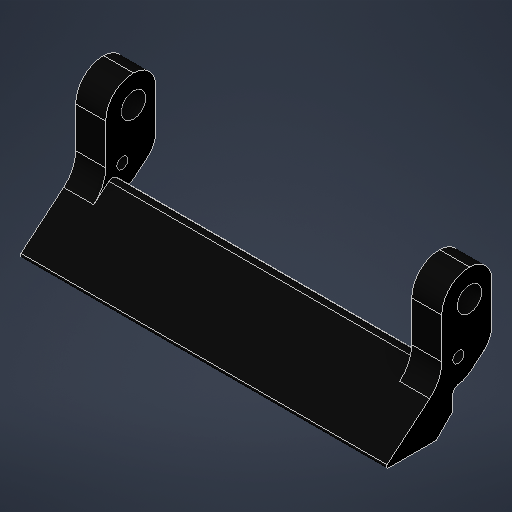
# Autodesk Inventor part: Schaufel
Saved by Autodesk Inventor 2025.2 (Build 292293000, 293)
## iProperties
Part Number: Schaufel
Material: Aluminium 6061
Document SubType Name: Modeling
Designer: rYan
Mass: 10.967 g
Surface Area: 30.2735 cm^2
Volume: 4.06184 cm^3
Density: 2.7 g/cm^3
Appearance: Vorgabe
Author: rYan
Autodesk Inventor part; units mm, degrees
ref_plane "YZ Plane" through (0, 0, 0) normal (1, 0, 0) x (0, 1, 0)
ref_plane "XZ Plane" through (0, 0, 0) normal (0, 1, 0) x (-1, 0, 0)
ref_plane "XY Plane" through (0, 0, 0) normal (0, 0, 1) x (1, 0, 0)
sketch "Skizze1" plane through (0, 0, 0) normal (1, 0, 0) x (0, 1, 0)
  line L0 (-4.1616, 7.0772) -> (-12, 0.5)
  line L1 (-12, 0) -> (-3, 0)
  line L2 (-12, 0.5) -> (-12, 0)
  line L3 (0, 5) -> (8, 11.7128)
  circle A0 centre (3, 19) radius 0.5
  line L4 (-2, 11.7128) -> (-2, 24)
  line L5 (-2, 24) -> (8, 24)
  line L6 (8, 24) -> (8, 11.7128)
  line L7 (0, 3) -> (-3, 0)
  line L8 (8, 11.7128) -> (-2, 11.7128) construction
  arc A1 (-4.1616, 7.0772) -> (-2, 11.7128) centre (-8.0514, 11.7128) ccw
  line L9 (0, 5) -> (0, 3)
  line L10 (3, 19) -> (3, 0) construction
  point P0 (0, 0)
  dimension "d40" = 0.5
  dimension "d44" = 1
  dimension "d59" = 10
  dimension "d60" = 45
  dimension "d61" = 5
  dimension "d63" = 40
  dimension "d78" = 3
  dimension "d79" = 12
  dimension "d80" = 0
  dimension "d81" = 19
  dimension "d82" = 5
  dimension "d83" = 3
  constraints: 22 end point, 5 vertical, 2 centre point, 2 horizontal, 2 point on circle, 2 tangent, 1 parallel, 1 perpendicular, 1 point on line, 1 other
  measures "d40" distance of L0.end L1.start
  measures "d44" diameter of A0
  measures "d59" distance of L4.end L5.end
  measures "d60" angle of L7 L1
  measures "d61" distance from line of L3.start L1
  measures "d63" angle of L0 L1
  measures "d78" distance of point (0, 0) L1.end
  measures "d79" distance from line of point (0, 0) L2
  measures "d80" distance from line of point (0, 0) L9
  measures "d81" vertical distance of point (0, 0) L10.start
  measures "d82" distance from line of L5 L10.start
  measures "d83" horizontal distance of point (0, 0) L10.start
extrude "Extrusion1" add sketch "Skizze1" along normal mid plane 67
sketch "Skizze6" plane through (0, 0, 0) normal (0, 1, 0) x (-1, 0, 0)
  line L0 (33.5, 0.5) -> (-33.5, 0.5) projected
  line L1 (-33.5, 7.0772) -> (-33.5, 0.5) projected
  line L2 (33.5, 0.5) -> (33.5, 7.0772) projected
  line L3 (-27.5, 6) -> (27.5, 6)
  line L4 (27.5, 6) -> (27.5, 31)
  line L5 (27.5, 31) -> (-27.5, 31)
  line L6 (-27.5, 31) -> (-27.5, 6)
  line L7 (0, -6.2) -> (0, 37.2) projected
  line L8 (33.5, 0) -> (-33.5, 0) projected
  line L9 (-33.5, 0) -> (33.5, 0) projected
  point P0 (0, 0)
  point P1 (-33, 10)
  point P2 (33, 10)
  dimension "d45" = 6
  dimension "d46" = 25
  dimension "d50" = 6
  constraints: 8 end point, 2 parallel, 1 horizontal, 1 perpendicular, 3 other
  measures "d46" distance of L3.end L4.end
  measures "d50" distance between parallel lines of L8 L3
extrude "Extrusion4" cut sketch "Skizze6" along normal mid plane 16
sketch "Skizze3" plane through (-33.5, 0, 0) normal (-1, 0, 0) x (0, 0, 1)
  line L0 (0, -3) -> (0, -12) projected
  line L1 (0.5, -12) -> (7.0772, -4.1616) projected
  line L2 (0, -12) -> (0, 0) construction
  line L3 (0, 12) -> (0, -16) projected
  line L4 (0, -12) -> (0.5, -12) projected
  line L5 (11.7128, 8) -> (5, 0) projected
  line L6 (11.7128, -2) -> (24, -2) projected
  line L7 (24, -2) -> (24, 8) projected
  line L8 (24, 8) -> (11.7128, 8) projected
  circle A0 centre (19, 3) radius 0.5 projected
  line L9 (3, 0) -> (0, -3) projected
  arc A1 (11.7128, -2) -> (7.0772, -4.1616) centre (11.7128, -8.0514) ccw projected
  line L10 (5, 0) -> (3, 0) projected
  constraints: 1 coincident
hole "Bohrung1" at (-33.5, 3, 19) direction (1, 0, 0) diameter 4.4 end through all
sketch "Skizze4" plane through (-33.5, 0, 0) normal (-1, 0, 0) x (0, 0, 1)
  line L0 (0, 12) -> (0, -16) projected
  line L1 (-5.8, 0) -> (34.8, 0) projected
  point P0 (29, 0)
  point P1 (11, 1)
  dimension "d38" = 11
  dimension "d84" = 1
  measures "d38" distance from line of point (11, 1) L0
  measures "d84" distance from line of point (11, 1) L1
hole "Bohrung2" at (-33.5, 1, 11) direction (1, 0, 0) diameter 2 end through all
fillet "Rundung2" radius 5 6 edges at (30.5, -2, 24) (30.5, 8, 24) (-30.5, 8, 24) (-30.5, -2, 24) (30.5, 8, 11.7128) (-30.5, 8, 11.7128)
fillet "Rundung8" radius 0.36 2 edges at (0, -12, 0.5) (0, -12, 0)
sketch "Skizze7" plane through (-27.5, 1.1918, 6) normal (0, 0, 1) x (1, 0, 0)
  line L0 (0, 0) -> (55, 0) projected
  line L1 (0, 0) -> (0, -6.6371) projected
  line L2 (55, -6.6371) -> (0, -6.6371) projected
  line L3 (55, -6.6371) -> (55, 0) projected
  line L4 (-19.4, -1.1918) -> (74.4, -1.1918) projected
  point P0 (27.5, -1.1918)
  point P1 (0, -1.1918)
  point P2 (55, -1.1918)
extrude "Extrusion5" cut sketch "Skizze7" against normal through all contours L0 L3 L4 L1
sketch "Skizze8" plane through (-27.5, -5.4454, 6) normal (1, 0, 0) x (0, 0, -1)
  line L0 (-8.0443, 13.4454) -> (-13, 13.4454) projected
  line L1 (-10.5222, 13.4454) -> (-10.5222, 12.4454)
  line L2 (-10.5222, 12.4454) -> (-17.4656, 12.4454)
  line L3 (-17.4656, 12.4454) -> (-4.9838, 12.4454)
  line L4 (-4.9838, 12.4454) -> (-4.9838, 14.4351)
  line L5 (-4.9838, 14.4351) -> (-17.4656, 14.4351)
  line L6 (-17.4656, 14.4351) -> (-17.4656, 12.4454)
  point P0 (6, 5.4454)
  dimension "d90" = 1
  constraints: 12 end point, 2 parallel, 2 perpendicular, 1 horizontal, 1 midpoint, 1 vertical
  measures "d90" distance of L1.start L1.end
extrude "Extrusion6" cut sketch "Skizze8" along normal mid plane 200
fillet "Rundung10" radius 4 4 edges at (30.5, 7, 11.0443) (30.5, 7, 22.0001) (-30.5, 7, 22.0001) (-30.5, 7, 11.0443)
sketch "Skizze9" plane through (-27.5, -2, 19) normal (1, 0, 0) x (0, 0, -1)
  line L0 (9.3252, 7.5712) -> (14, 2) projected
  line L1 (14, 2) -> (14, 3)
  line L2 (14, 3) -> (12.8, 3)
  line L3 (12.8, 3) -> (14, 3)
  line L4 (14, 3) -> (14, 4.2192)
  line L5 (14, 4.2192) -> (12.8, 4.2192)
  line L6 (12.8, 4.2192) -> (12.8, 3)
  line L7 (12.3, 4.7192) -> (14.5, 4.7192)
  line L8 (14.5, 4.7192) -> (14.5, 2.5)
  line L9 (14.5, 2.5) -> (12.3, 2.5)
  line L10 (12.3, 2.5) -> (12.3, 4.7192)
  line L11 (12.3, 2.5) -> (12.3, 1.2569)
  line L12 (12.3, 1.2569) -> (14.6235, 1.2569)
  line L13 (12.3, 1.2569) -> (11.55, 1.2569)
  line L14 (11.55, 1.2569) -> (11.55, 4.7192)
  line L15 (11.55, 4.7192) -> (12.3, 4.7192)
  point P0 (19, 2)
  point P1 (13.5805, 2.5)
  point P2 (12.3, 4.026)
  point P3 (11.55, 4.45)
  point P4 (13.1609, 3)
  point P5 (14, 2.5)
  dimension "d95" = 1
  dimension "d96" = 1.2
  dimension "d97" = 0.5
  dimension "d103" = 0.75
  constraints: 30 end point, 6 perpendicular, 4 parallel, 2 horizontal, 2 vertical, 1 point on line, 3 other
  measures "d95" distance of L0.end L1.end
  measures "d96" distance of L1.end L2.end
  measures "d97" distance between parallel lines of L5 L7
  measures "d103" distance of L11.end L13.end
extrude "Extrusion7" cut sketch "Skizze9" along normal mid plane 200 contours L10 L7 L8 L9 L1 L4 L5 L6 L0 | L0 L6 L2 L9 L10 | L6 L5 L4 L2 L0 | L0 L2 L6 | L2 L1 L9 L0 | L9 L1 L0
fillet "Rundung12" radius 4 2 edges at (30.5, 2.026, 6.7) (-30.5, 2.026, 6.7)
sketch "Skizze16" plane through (-27.5, 0, 6) normal (0, 0, 1) x (1, 0, 0)
  line L0 (27.5, 0) -> (27.5, -5.4454)
  line L1 (55, -5.4454) -> (0, -5.4454) projected
  line L2 (27.5, -5.4454) -> (27.5, -26.9454)
  circle A0 centre (27.5, -26.9454) radius 21.5
  circle A1 centre (27.5, -26.9454) radius 24.5
  line L3 (0, -5.4454) -> (0, 0)
  line L4 (-6, 0) -> (61, 0) projected
  line L5 (0, 0) -> (55, 0)
  line L6 (55, 0) -> (55, -5.4454)
  line L7 (55, -5.4454) -> (0, -5.4454)
  line L8 (0, -5.4454) -> (0, 0)
  point P0 (15.7527, -5.4454)
  point P1 (39.2473, -5.4454)
  point P2 (55, 0)
  dimension "d122" = 21.5
  dimension "d123" = 3
  constraints: 14 end point, 2 parallel, 2 point on line, 1 centre point, 1 coincident, 1 horizontal, 1 midpoint, 1 perpendicular, 1 vertical, 1 vertical alignment, 2 other
  measures "d122" distance of L0.end L2.end
extrude "Extrusion11" add sketch "Skizze16" along normal blind 5 contours L4 L6 L1 A1 L0 | L0 A1 L1 L3 L4 | A1 L1 L0 | L0 L1 A1
sketch "Skizze18" plane through (27.5, -5.4454, 11) normal (1, 0, 0) x (0, 0, -1)
  line L0 (10.3642, -6.3928) -> (3.9228, 1.2837) projected
  line L1 (10.3642, -6.3928) -> (0, 5.9588)
  line L2 (0, 0) -> (0, 3.4032) projected
  line L3 (0, 5.9588) -> (0, 0)
  line L4 (0, 0) -> (5, 0)
  point P0 (11, 5.4454)
  point P1 (5, 0)
  constraints: 6 end point, 2 collinear, 1 perpendicular, 1 point on line
extrude "Extrusion12" cut sketch "Skizze18" against normal up to surface (55 mm away)
sketch "Skizze19" plane through (27.5, -2, 11.7128) normal (-1, 0, 0) x (0, 0, 1)
  circle A0 centre (-0.7128, 3) radius 1 projected
  circle A1 centre (-0.7128, 3) radius 2
  point P0 (-11.7128, 2)
  dimension "d131" = 4
  constraints: 1 centre point, 1 coincident
  measures "d131" diameter of A1
extrude "Extrusion13" cut sketch "Skizze19" along normal up to surface (55 mm away) contours A0 | A1
sketch "Skizze22" plane through (33.5, 0, 0) normal (1, 0, 0) x (0, 0, -1)
  line L0 (0, -3) -> (-3, 0) projected
  line L1 (-5.4195, 0.5) -> (-6.7, 0.5) projected
  line L2 (-3, 0) -> (-6.7, 0)
  line L3 (-6.7, 0) -> (-6.7, 0.5)
  line L4 (-6.7, 0.5) -> (-3, 0.5)
  line L5 (-3, 0.5) -> (-3, 0)
  point P0 (0, 0)
  point P1 (-5.4195, 0.5)
  constraints: 8 end point, 2 parallel, 1 horizontal, 1 perpendicular
extrude "Extrusion14" cut sketch "Skizze22" against normal up to surface (67 mm away)
fillet "Rundung22" radius 1 2 edges at (30.5, 0, 6.7) (-30.5, 0, 6.7)
sketch "Skizze23" plane through (-33.5, -2, 11.7128) normal (0, -1, 0) x (1, 0, 0)
  line L0 (0, 8.2872) -> (0, 12.2872) projected
  line L1 (0, 12.2872) -> (67, 12.2872)
  line L2 (67, 12.2872) -> (67, -11.7128)
  line L3 (67, -11.7128) -> (0, -11.7128)
  line L4 (0, -11.7128) -> (0, 12.2872)
  line L5 (66.4, 11.6872) -> (0.6, 11.6872)
  line L6 (0.6, 11.6872) -> (0.6, -11.1128)
  line L7 (0.6, -11.1128) -> (66.4, -11.1128)
  line L8 (66.4, -11.1128) -> (66.4, 11.6872)
  line L9 (66.4, 11.6872) -> (66.4, 12.2872)
  line L10 (66.4, -11.1128) -> (66.4, -11.7128)
  line L11 (0.6, -11.1128) -> (0.6, -11.7128)
  line L12 (0.6, 11.6872) -> (0.6, 12.2872)
  dimension "d146" = 0.6
  constraints: 24 end point, 5 perpendicular, 5 point on line, 4 parallel, 1 horizontal, 3 other
  measures "d146" distance between parallel lines of L1 L5
extrude "Extrusion15" cut sketch "Skizze23" along normal mid plane 100 contours L0 L1 L12 L6 L11 L3 L4 | L1 L2 L3 L10 L8 L9
fillet "Rundung23" radius 1 1 edges at (0, -0.7143, 9.9698)
